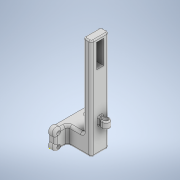
# Autodesk Inventor part: Soporte_Sensor_Fin_Carrera
Saved by Autodesk Inventor 2021 (Build 250183000, 183)
## iProperties
Created: 2021-04-15
Part Number: Soporte_Sensor_Fin_Carrera
Material: Genérico
Document SubType Name: Modeling
Designer: Joaquín
Density: 1 g/cm^3
Appearance: Valor por defecto
Author: Joaquín
Autodesk Inventor part; units mm, degrees
ref_plane "YZ Plane" through (0, 0, 0) normal (1, 0, 0) x (0, 1, 0)
ref_plane "XZ Plane" through (0, 0, 0) normal (0, 1, 0) x (-1, 0, 0)
ref_plane "XY Plane" through (0, 0, 0) normal (0, 0, 1) x (1, 0, 0)
sketch "Boceto1" plane through (0, 0, 0) normal (1, 0, 0) x (0, 1, 0)
  point P0 (0, 0)
sketch "Boceto2" plane through (0, 0, 0) normal (1, 0, 0) x (0, 1, 0)
  line L0 (5, 0) -> (10, 0)
  line L1 (15, -5) -> (15, -30)
  line L2 (10, -35) -> (5, -35)
  line L3 (0, -30) -> (0, -5)
  circle A0 centre (2.5, -32.5) radius 1.5
  circle A1 centre (12.5, -32.5) radius 1.5
  circle A2 centre (2.5, -2.5) radius 1.5
  circle A3 centre (12.5, -2.5) radius 1.5
  arc A4 (0, -30) -> (5, -35) centre (2.5, -32.5) ccw
  arc A5 (5, 0) -> (0, -5) centre (2.5, -2.5) ccw
  arc A6 (15, -5) -> (10, 0) centre (12.5, -2.5) ccw
  arc A7 (10, -35) -> (15, -30) centre (12.5, -32.5) ccw
  point P0 (0, 0)
  constraints: 9 point on circle, 8 centre point, 8 end point, 4 coincident, 2 vertical, 1 horizontal, 1 perpendicular
extrude "Extrusión1" add sketch "Boceto2" along normal blind 5
sketch "Boceto3" plane through (5, 0, 0) normal (1, 0, 0) x (0, 0, -1)
  line L0 (5, 0) -> (30, 0) projected
  arc A0 (5, 15) -> (0, 10) centre (2.5, 12.5) ccw projected
  line L1 (30, 15) -> (5, 15) projected
  line L2 (25, 7.5) -> (25, 0)
  line L3 (25, 7.5) -> (25, 15)
  line L4 (25, 15) -> (10, 15)
  line L5 (10, 15) -> (10, 0)
  line L6 (25, 0) -> (10, 0)
  point P0 (0, 0)
  constraints: 10 end point, 4 point on line, 3 perpendicular, 1 collinear
extrude "Extrusión2" add sketch "Boceto3" along normal blind 20
sketch "Boceto4" plane through (0, 15, -5) normal (0, 1, 0) x (1, 0, 0)
  line L0 (25, 20) -> (25, 5) projected
  line L1 (25, 20) -> (18, 20)
  line L2 (5, 20) -> (25, 20) projected
  line L3 (18, 20) -> (18, 5)
  line L4 (5, 5) -> (25, 5) projected
  line L5 (25, 5) -> (18, 5)
  line L6 (25, 5) -> (25, 20)
  point P0 (0, -5)
  constraints: 8 end point, 2 collinear, 2 point on line, 1 perpendicular
extrude "Extrusión3" add sketch "Boceto4" along normal blind 70
fillet "Empalme1" radius 2 16 edges at (5, 0, -27.5) (5, 15, -27.5) (5, 7.5, -25) (11.5, 15, -25) (15, 0, -25) (25, 0, -17.5) (18, 15, -17.5) (18, 50, -25) (25, 42.5, -25) (25, 42.5, -10) (15, 0, -10) (11.5, 15, -10) (18, 50, -10) (5, 7.5, -10) (5, 0, -7.5) (5, 15, -7.5)
fillet "Empalme2" radius 2 10 edges at (5, 15, 0) (5, 14.0811, -5.6623) (5, 7.5, 0) (5, 0.9189, -5.6623) (5, 0, 0) (5, 7.5, -35) (5, 0.9189, -29.3377) (5, 0, -35) (5, 14.0811, -29.3377) (5, 15, -35)
sketch "Boceto5" plane through (25, 0, 0) normal (1, 0, 0) x (0, 0, -1)
  line L0 (14.5, 82.5) -> (14.5, 62.5)
  line L1 (14.5, 62.5) -> (20.5, 62.5)
  line L2 (20.5, 62.5) -> (20.5, 82.5)
  line L3 (20.5, 82.5) -> (14.5, 82.5)
  point P0 (0, 0)
  point P1 (23, 85)
  point P2 (12, 85)
  constraints: 8 end point, 2 perpendicular
extrude "Extrusión4" cut sketch "Boceto5" against normal blind 70
fillet "Empalme3" radius 1 8 edges at (25, 85, -17.5) (24.4142, 85, -24.4142) (21.5, 85, -25) (18.5858, 85, -24.4142) (18, 85, -17.5) (18.5858, 85, -10.5858) (21.5, 85, -10) (24.4142, 85, -10.5858)
sketch "Boceto6" plane through (25, 0, 0) normal (1, 0, 0) x (0, 0, -1)
  line L0 (27, 15) -> (23, 15) projected
  arc A0 (12, 15) -> (10, 13) centre (12, 13) ccw projected
  line L1 (23, 84) -> (23, 2) projected
  arc A1 (25, 13) -> (23, 15) centre (23, 13) ccw projected
  line L2 (17.5, 21.5263) -> (14.5, 21.5263)
  line L3 (14.5, 21.5263) -> (14.5, 27.5263)
  line L4 (14.5, 27.5263) -> (20.5, 27.5263)
  line L5 (20.5, 27.5263) -> (20.5, 21.5263)
  line L6 (20.5, 21.5263) -> (17.5, 21.5263)
  point P0 (0, 0)
  constraints: 10 end point, 2 perpendicular, 1 collinear, 1 point on line
extrude "Extrusión5" add sketch "Boceto6" along normal blind 10
sketch "Boceto7" plane through (25, 27.5263, -14.5) normal (0, 1, 0) x (1, 0, 0)
  line L0 (0, 6) -> (10, 6) projected
  line L1 (0, 0) -> (10, 0) projected
  line L2 (10, 6) -> (10, 0) projected
  circle A0 centre (4.8038, 3) radius 3
  line L3 (4.8038, 6) -> (10, 6)
  line L4 (10, 0) -> (4.8038, 0)
  line L5 (10, 0) -> (10, 6)
  point P0 (-25, -14.5)
  constraints: 7 end point, 2 point on circle, 2 point on line, 2 tangent, 1 centre point, 1 collinear, 1 vertical
extrude "Extrusión6" cut sketch "Boceto7" against normal blind 10 contours L0 L2 L1 A0
sketch "Boceto8" plane through (25, 27.5263, -14.5) normal (0, 1, 0) x (1, 0, 0)
  arc A0 (4.8038, 0) -> (4.8038, 6) centre (4.8038, 3) ccw projected
  circle A1 centre (4.8038, 3) radius 2
  line L0 (0, 0) -> (0, 6) projected
  line L1 (0, 6) -> (0, 4.5)
  line L2 (0, 0) -> (0, 1.5)
  arc A2 (0, 4.5) -> (2.8038, 6) centre (0.2019, 7.4932) ccw
  line L3 (0, 0) -> (4.8038, 0) projected
  arc A3 (2.8038, 0) -> (0, 1.5) centre (0.2019, -1.4932) ccw
  line L4 (0, 6) -> (4.8038, 6) projected
  line L5 (2.8038, 6) -> (0, 6)
  line L6 (2.8038, 0) -> (0, 0)
  point P0 (-25, -14.5)
  dimension "d39" = 4
  dimension "d40" = 1.5
  dimension "d41" = 1.5
  dimension "d42" = 3
  dimension "d43" = 3
  constraints: 8 end point, 4 point on circle, 3 centre point, 3 point on line, 1 coincident, 1 collinear
  measures "d39" diameter of A1
  measures "d40" distance of L0.end L1.end
  measures "d41" distance of L0.start L2.end
  measures "d42" radius of A2
  measures "d43" radius of A3
extrude "Extrusión7" cut sketch "Boceto8" against normal blind 10 contours L3 L0 A3 | A2 L0 L4 | A1
fillet "Empalme4" radius 1 16 edges at (25, 24.5263, -19) (25, 27.5263, -17.5) (25, 24.5263, -16) (25, 21.5263, -17.5) (26.617, 21.5263, -15.652) (26.617, 27.5263, -15.652) (26.617, 27.5263, -19.348) (26.617, 21.5263, -19.348) (28.8038, 21.5263, -14.5) (28.8038, 21.5263, -20.5) (32.8038, 21.5263, -17.5) (28.8038, 27.5263, -20.5) (28.8038, 27.5263, -14.5) (32.8038, 27.5263, -17.5) (27.8038, 24.5263, -20.5) (27.8038, 24.5263, -14.5)
